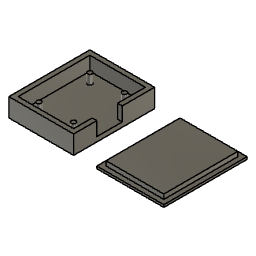
Wired sensor box (Autodesk Fusion 360 design; units mm, degrees)
Autodesk Fusion 360 part; units mm, degrees
sketch "Sketch1" plane through (0, 0, 0) normal (0, 0, 1) x (1, 0, 0)
  line L0 (-28, 35) -> (0, 35)
  line L1 (0, 35) -> (0, 0)
  line L2 (0, 0) -> (-28, 0)
  line L3 (-28, 0) -> (-28, 35)
  circle A0 centre (-21.5, 28.5) radius 1
  circle A1 centre (-6.5, 28.5) radius 1
  circle A2 centre (-21.5, 6.5) radius 1
  circle A3 centre (-6.5, 6.5) radius 1
  line L4 (-32, 28.5) -> (12, 28.5) construction
  line L5 (-6.5, 33) -> (-6.5, -2) construction
  line L6 (-28, 6.5) -> (6, 6.5) construction
  line L7 (-21.5, 33) -> (-21.5, -2) construction
  line L8 (-26, 33) -> (-2, 33)
  line L9 (-2, 33) -> (-2, 2)
  line L10 (-2, 2) -> (-26, 2)
  line L11 (-26, 2) -> (-26, 33)
  point P0 (-21.5, 25)
  dimension "d1" = 35
  dimension "d2" = 28
  dimension "d3" = 2
  dimension "d4" = 15
  dimension "d5" = 22
  dimension "d7" = 6.5
  dimension "d8" = 6.5
  dimension "d13" = 2
  dimension "d14" = 2
  dimension "d15" = 2
  dimension "d16" = 2
  constraint horizontal L0
  constraint vertical L1
  constraint horizontal L2
  constraint vertical L3
  constraint coincident L1.end L2.start
  constraint equal A1 A3
  constraint equal A0 A2
  constraint equal A2 A3
  constraint horizontal L4
  constraint perpendicular L2 L5
  constraint perpendicular L1 L6
  constraint perpendicular L0 L7
  constraint coincident A1.centre L5
  constraint coincident P0 L7
  constraint coincident A0.centre L4
  constraint coincident A0.centre L7
  constraint coincident A2.centre L6
  constraint coincident A2.centre L7
  constraint coincident A3.centre L5
  constraint coincident A3.centre L6
  constraint coincident A1.centre L4
  constraint horizontal L8
  constraint vertical L9
  constraint horizontal L10
  constraint vertical L11
  measures "d1" distance of L0.end L1.end
  measures "d2" distance of L0.start L0.end
  measures "d3" diameter of A0
  measures "d4" distance of L5 L7
  measures "d5" distance of L4 L6
  measures "d7" distance of L0 L4
  measures "d8" distance of L3 L7
  measures "d13" distance of L1 L9
  measures "d14" distance of L0 L8
  measures "d15" distance of L2 L10
  measures "d16" distance of L3 L11
extrude "Extrude1" add sketch "Sketch1" along normal blind 2 contours L0 L1 L2 L3 | L8 L9 L10 L11 makes body 1
extrude "Extrude2" add sketch "Sketch1" along normal blind 6 contours A0 | A1 | A2 | A3 bodies 1
extrude "Extrude3" cut sketch "Sketch1" along normal blind 8 contours L0 L1 L2 L3 bodies 1
extrude "Extrude4" add sketch "Sketch1" along normal blind 8 contours L0 L1 L2 L3 bodies 1
sketch "Sketch3" plane through (0, 0, 0) normal (0, 0, 1) x (1, 0, 0)
  line L0 (10, 36) -> (39, 36)
  line L1 (39, 36) -> (39, 0)
  line L2 (39, 0) -> (10, 0)
  line L3 (10, 0) -> (10, 36)
  line L4 (12, 34) -> (37, 34)
  line L5 (37, 34) -> (37, 2)
  line L6 (37, 2) -> (12, 2)
  line L7 (12, 2) -> (12, 34)
  line L8 (-40, 0) -> (50, 0) construction
  point P0 (-28, 0)
  dimension "d21" = 29
  dimension "d22" = 36
  dimension "d23" = 2
  dimension "d24" = 2
  dimension "d25" = 2
  dimension "d26" = 2
  constraint horizontal L0
  constraint vertical L1
  constraint horizontal L2
  constraint vertical L3
  constraint horizontal L4
  constraint vertical L5
  constraint horizontal L6
  constraint vertical L7
  constraint perpendicular L5 L8
  constraint coincident L8 P0
  constraint coincident L2.end L8
  measures "d21" distance of L0.start L0.end
  measures "d22" distance of L0.end L1.end
  measures "d23" distance of L0 L4
  measures "d24" distance of L1 L5
  measures "d25" distance of L2 L6
  measures "d26" distance of L3 L7
extrude "Extrude5" add sketch "Sketch3" along normal blind 1 separate body makes body 2
extrude "Extrude6" add sketch "Sketch3" along normal blind 3 contours L4 L5 L6 L7 bodies 2
sketch "Sketch4" plane through (0, 0, 0) normal (1, 0, 0) x (0, 1, 0)
  line L0 (0, 0) -> (35, 0)
  line L1 (35, 0) -> (35, 8)
  line L2 (35, 8) -> (0, 8)
  line L3 (0, 8) -> (0, 0)
  line L4 (10, 8) -> (21, 8)
  line L5 (21, 8) -> (21, 2)
  line L6 (21, 2) -> (10, 2)
  line L7 (10, 2) -> (10, 8)
  dimension "d31" = 6
  dimension "d32" = 11
  dimension "d33" = 10
  constraint horizontal L4
  constraint vertical L5
  constraint horizontal L6
  constraint vertical L7
  constraint coincident L2 L4.start
  measures "d31" distance of L4.start L6.end
  measures "d32" distance of L5.end L6.end
  measures "d33" distance of L3 L7
extrude "Extrude7" cut sketch "Sketch4" against normal blind 3 contours L2 L4 L5 L6 L7 bodies 1
equation "d7 = ( d1 - d5 ) / 2"
equation "d8 = ( d2 - d4 ) / 2"
